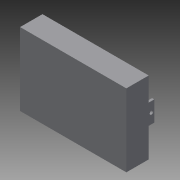
# Autodesk Inventor part: RESONATORCHAMBER
Saved by Autodesk Inventor 2013 (Build 170138000, 138)
## iProperties
Created: 2013-06-23
Part Number: RESONATORCHAMBER
Material: Generic
Document SubType Name: Modeling
Designer: Virtual
Density: 1 g/cm^3
Author: Virtual
Autodesk Inventor part; units mm, degrees
ref_plane "YZ Plane" through (0, 0, 0) normal (1, 0, 0) x (0, 1, 0)
ref_plane "XZ Plane" through (0, 0, 0) normal (0, 1, 0) x (-1, 0, 0)
sketch "Sketch1" plane through (0, 0, 0) normal (0, 1, 0) x (-1, 0, 0)
  line L0 (0, 0) -> (95, 0)
  line L1 (95, 0) -> (95, 65)
  line L2 (95, 65) -> (0, 65)
  line L3 (0, 65) -> (0, 0)
  constraints: 8 end point, 2 parallel, 1 horizontal, 1 perpendicular
extrude "Extrusion1" add sketch "Sketch1" along normal blind 20
sketch "Sketch2" plane through (0, 20, 0) normal (0, 1, 0) x (1, 0, 0)
  line L0 (-5, -5) -> (-90, -5)
  line L1 (-90, -5) -> (-90, -60)
  line L2 (-90, -60) -> (-5, -60)
  line L3 (-5, -60) -> (-5, -5)
  constraints: 8 end point, 2 parallel, 1 horizontal, 1 perpendicular
extrude "Extrusion2" cut sketch "Sketch2" against normal blind 15
sketch "Sketch5" plane through (-90, 20, 60) normal (1, 0, 0) x (0, 0, -1)
  line L0 (0, -15) -> (55, -15) projected
  line L1 (21, -4) -> (39, -4)
  line L2 (39, -4) -> (39, 10)
  line L3 (39, 10) -> (21, 10)
  line L4 (21, 10) -> (21, -4)
  point P0 (60, -20)
  point P1 (60, 0)
  dimension "d12" = 18
  dimension "d13" = 14
  dimension "d15" = 21
  dimension "d16" = 11
  constraints: 8 end point, 2 parallel, 1 horizontal, 1 perpendicular
  measures "d12" distance of L3.end L2.end
  measures "d13" distance of L2.end L1.end
  measures "d15" distance from line of L2 point (60, 0)
  measures "d16" distance between parallel lines of L0 L1
extrude "Extrusion3" add sketch "Sketch5" along normal blind 2
ref_plane "Work Plane1" through (-47.5, 5, 60) normal (1, 0, 0) x (0, 0, -1)
mirror "Mirror1" about plane through (-47.5, 5, 60) normal (1, 0, 0) of "Extrusion3"
sketch "Sketch7" plane through (-5, 20, 21) normal (1, 0, 0) x (0, 0, -1)
  line L0 (0, 10) -> (-18, 10) projected
  line L1 (-18, 10) -> (-18, 0) projected
  point P0 (21, -20)
  point P1 (-9, 7.5)
  dimension "d19" = 9
  dimension "d20" = 2.5
  measures "d19" distance from line of L1 point (-9, 7.5)
  measures "d20" distance from line of L0 point (-9, 7.5)
hole "Hole2" at (-5, 27.5, 30) direction (-1, 0, 0) diameter 3.25 end through all
body "Solid1"
